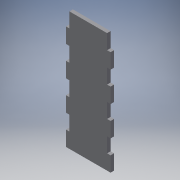
# Autodesk Inventor part: WallBend
Saved by Autodesk Inventor 2017 (Build 210142000, 142)
## iProperties
Created: 2017-03-28
Part Number: WallBend
Material: Generic
Document SubType Name: Modeling
Designer: hoeflinc
Density: 1 g/cm^3
Appearance: Default
Quantity: 1
Author: hoeflinc
Autodesk Inventor part; units mm, degrees
ref_plane "YZ Plane" through (0, 0, 0) normal (1, 0, 0) x (0, 1, 0)
ref_plane "XZ Plane" through (0, 0, 0) normal (0, 1, 0) x (-1, 0, 0)
ref_plane "XY Plane" through (0, 0, 0) normal (0, 0, 1) x (1, 0, 0)
sketch "Sketch1" plane through (0, 0, 0) normal (0, 0, 1) x (1, 0, 0)
  line L0 (0, 0) -> (38.1, 0)
  line L1 (38.1, 0) -> (38.1, 101.6)
  line L2 (38.1, 101.6) -> (0, 101.6)
  line L3 (0, 101.6) -> (0, 0)
  dimension "d0" = 38.1
  dimension "d1" = 101.6
  constraints: 8 end point, 2 parallel, 1 horizontal, 1 perpendicular
  measures "d0" distance of L0.start L0.end
  measures "d1" distance of L2.end L0.start
extrude "Extrusion1" add sketch "Sketch1" along normal blind 3
sketch "Sketch2" plane through (0, 0, 3) normal (0, 0, 1) x (1, 0, 0)
  line L0 (0, 0) -> (38.1, 0) projected
  line L1 (38.1, 0) -> (38.1, 101.6) projected
  line L2 (38.1, 101.6) -> (0, 101.6) projected
  line L3 (0, 101.6) -> (0, 0) projected
  line L4 (38.1, 12.8016) -> (35.1, 12.8016)
  line L5 (35.1, 12.8016) -> (35.1, 25.2984)
  line L6 (35.1, 25.2984) -> (38.1, 25.2984)
  line L7 (38.1, 25.2984) -> (38.1, 12.8016)
  line L8 (35.1, 38.2016) -> (35.1, 50.6984)
  line L9 (35.1, 50.6984) -> (38.1, 50.6984)
  line L10 (38.1, 38.2016) -> (35.1, 38.2016)
  line L11 (38.1, 50.6984) -> (38.1, 38.2016)
  line L12 (35.1, 63.6016) -> (35.1, 76.0984)
  line L13 (35.1, 76.0984) -> (38.1, 76.0984)
  line L14 (38.1, 63.6016) -> (35.1, 63.6016)
  line L15 (38.1, 76.0984) -> (38.1, 63.6016)
  line L16 (35.1, 89.0016) -> (35.1, 101.4984)
  line L17 (35.1, 101.4984) -> (38.1, 101.4984)
  line L18 (38.1, 89.0016) -> (35.1, 89.0016)
  line L19 (38.1, 101.4984) -> (38.1, 89.0016)
  line L20 (0, 0) -> (38.1, 0) construction
  line L21 (19.05, 0) -> (19.05, 101.6) construction
  line L22 (0, 12.8016) -> (3, 12.8016)
  line L23 (3, 12.8016) -> (3, 25.2984)
  line L24 (3, 25.2984) -> (0, 25.2984)
  line L25 (3, 38.2016) -> (3, 50.6984)
  line L26 (3, 50.6984) -> (0, 50.6984)
  line L27 (0, 38.2016) -> (3, 38.2016)
  line L28 (3, 63.6016) -> (3, 76.0984)
  line L29 (3, 76.0984) -> (0, 76.0984)
  line L30 (0, 63.6016) -> (3, 63.6016)
  line L31 (0, 76.0984) -> (0, 63.6016)
  line L32 (3, 89.0016) -> (3, 101.4984)
  line L33 (3, 101.4984) -> (0, 101.4984)
  line L34 (0, 89.0016) -> (3, 89.0016)
  line L35 (0, 101.4984) -> (0, 89.0016)
  line L36 (0, 38.2016) -> (0, 50.6984)
  line L37 (0, 101.6) -> (0, 0) projected
  line L38 (0, 12.8016) -> (0, 25.2984)
  dimension "d4" = 12.4968
  dimension "d5" = 12.8016
  dimension "d6" = 3
  dimension "d9" = 25.4
  constraints: 66 end point, 16 symmetric about line, 2 collinear, 2 midpoint, 2 parallel, 1 horizontal, 1 perpendicular, 1 point on line, 1 vertical, 24 other
  measures "d4" distance between parallel lines of L6 L4
  measures "d5" distance between parallel lines of L4 L0
  measures "d6" distance between parallel lines of L1 L5
  measures "d9" distance of L4.end L8.start
extrude "Extrusion2" cut sketch "Sketch2" against normal blind 3 contours L3 L24 L23 L22 | L4 L5 L6 L1 | L3 L26 L25 L27 | L10 L8 L9 L1 | L3 L29 L28 L30 | L14 L12 L13 L1 | L3 L33 L32 L34 | L18 L16 L17 L1
sketch "Sketch3" plane through (0, 0, 3) normal (0, 0, 1) x (1, 0, 0)
  line L0 (35.1, 76.0984) -> (38.1, 76.0984) projected
  line L1 (38.1, 76.0984) -> (38.1, 89.0016) projected
  line L2 (38.1, 89.0016) -> (35.1, 89.0016) projected
  line L3 (35.1, 89.0016) -> (35.1, 101.4984) projected
  line L4 (35.1, 101.4984) -> (38.1, 101.4984) projected
  line L5 (38.1, 101.4984) -> (38.1, 101.6) projected
  line L6 (38.1, 101.6) -> (0, 101.6) projected
  line L7 (0, 101.6) -> (0, 101.4984) projected
  line L8 (0, 0) -> (38.1, 0) projected
  line L9 (38.1, 0) -> (38.1, 12.8016) projected
  line L10 (38.1, 12.8016) -> (35.1, 12.8016) projected
  line L11 (35.1, 12.8016) -> (35.1, 25.2984) projected
  line L12 (35.1, 25.2984) -> (38.1, 25.2984) projected
  line L13 (38.1, 25.2984) -> (38.1, 38.2016) projected
  line L14 (38.1, 38.2016) -> (35.1, 38.2016) projected
  line L15 (35.1, 38.2016) -> (35.1, 50.6984) projected
  line L16 (35.1, 50.6984) -> (38.1, 50.6984) projected
  line L17 (38.1, 50.6984) -> (38.1, 63.6016) projected
  line L18 (38.1, 63.6016) -> (35.1, 63.6016) projected
  line L19 (35.1, 63.6016) -> (35.1, 76.0984) projected
  line L20 (38.1, 101.4984) -> (35.1, 101.4984) projected
  line L21 (38.1, 101.6) -> (35.1, 101.6)
  line L22 (35.1, 101.6) -> (35.1, 101.4984)
  line L23 (35.1, 101.4984) -> (38.1, 101.4984)
  line L24 (38.1, 101.4984) -> (38.1, 101.6)
  line L25 (3, 38.2016) -> (0, 38.2016) projected
  line L26 (0, 38.2016) -> (0, 25.2984) projected
  line L27 (0, 25.2984) -> (3, 25.2984) projected
  line L28 (3, 25.2984) -> (3, 12.8016) projected
  line L29 (3, 12.8016) -> (0, 12.8016) projected
  line L30 (0, 12.8016) -> (0, 0) projected
  line L31 (0, 101.4984) -> (3, 101.4984) projected
  line L32 (3, 101.4984) -> (3, 89.0016) projected
  line L33 (3, 89.0016) -> (0, 89.0016) projected
  line L34 (0, 89.0016) -> (0, 76.0984) projected
  line L35 (0, 76.0984) -> (3, 76.0984) projected
  line L36 (3, 76.0984) -> (3, 63.6016) projected
  line L37 (3, 63.6016) -> (0, 63.6016) projected
  line L38 (0, 63.6016) -> (0, 50.6984) projected
  line L39 (0, 50.6984) -> (3, 50.6984) projected
  line L40 (3, 50.6984) -> (3, 38.2016) projected
  line L41 (3, 101.4984) -> (0, 101.4984) projected
  line L42 (0, 101.6) -> (3, 101.6)
  line L43 (3, 101.6) -> (3, 101.4984)
  line L44 (3, 101.4984) -> (0, 101.4984)
  line L45 (0, 101.4984) -> (0, 101.6)
  constraints: 16 end point, 4 parallel, 2 horizontal, 2 perpendicular
extrude "Extrusion3" cut sketch "Sketch3" against normal blind 3 contours L22 L6 L5 L4 | L43 L31 L7 L6
body "Solid1"
